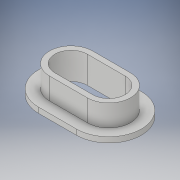
# Autodesk Inventor part: Flanec_podProvoda
Saved by Autodesk Inventor 2017 (Build 210142000, 142)
## iProperties
Part Number: Flanec_podProvoda
Material: Типовые
Document SubType Name: Modeling
Designer: Тетяна
Density: 1 g/cm^3
Appearance: По умолчанию
Author: Тетяна
Autodesk Inventor part; units mm, degrees
ref_plane "YZ Plane" through (0, 0, 0) normal (1, 0, 0) x (0, 1, 0)
ref_plane "XZ Plane" through (0, 0, 0) normal (0, 1, 0) x (-1, 0, 0)
ref_plane "XY Plane" through (0, 0, 0) normal (0, 0, 1) x (1, 0, 0)
sketch "Эскиз1" plane through (0, 0, 0) normal (0, 1, 0) x (-1, 0, 0)
  line L0 (0, 0) -> (-7, 0) construction
  line L1 (0, 4) -> (-7, 4)
  line L2 (-7, -4) -> (0, -4)
  arc A0 (0, -4) -> (0, 4) centre (0, 0) ccw
  arc A1 (-7, 4) -> (-7, -4) centre (-7, 0) ccw
  point P0 (-3.5, 0)
  dimension "d0" = 7
  dimension "d1" = 8
  constraints: 8 end point, 4 point on circle, 4 tangent, 2 centre point, 1 horizontal, 1 midpoint, 1 parallel
  measures "d0" distance of L0.start L0.end
  measures "d1" diameter of A1
extrude "Выдавливание1" add sketch "Эскиз1" along normal blind 5
sketch "Эскиз2" plane through (0, 0, 0) normal (0, -1, 0) x (1, 0, 0)
  line L0 (0, 4) -> (7, 4) projected
  arc A0 (0, 4) -> (0, -4) centre (0, 0) ccw projected
  line L1 (7, -4) -> (0, -4) projected
  arc A1 (7, -4) -> (7, 4) centre (7, 0) ccw projected
  arc A2 (0, 6) -> (0, -6) centre (0, 0) ccw
  line L2 (0, 6) -> (7, 6)
  arc A3 (7, -6) -> (7, 6) centre (7, 0) ccw
  line L3 (7, -6) -> (0, -6)
  dimension "d4" = 2
  constraints: 4 end point, 4 point on circle, 2 centre point, 3 other
  measures "d4" radial gap between concentric circles of A0 A2
extrude "Выдавливание2" add sketch "Эскиз2" against normal blind 1
sketch "Эскиз3" plane through (0, 5, 0) normal (0, 1, 0) x (1, 0, 0)
  line L0 (0, -4) -> (7, -4) projected
  arc A0 (7, -4) -> (7, 4) centre (7, 0) ccw projected
  line L1 (7, 4) -> (0, 4) projected
  arc A1 (0, 4) -> (0, -4) centre (0, 0) ccw projected
  line L2 (0, 3) -> (7, 3)
  arc A2 (7, -3) -> (7, 3) centre (7, 0) ccw
  line L3 (7, -3) -> (0, -3)
  arc A3 (0, 3) -> (0, -3) centre (0, 0) ccw
  dimension "d7" = 1
  constraints: 4 end point, 4 point on circle, 2 centre point, 3 other
  measures "d7" distance between parallel lines of L1 L2
extrude "Выдавливание3" cut sketch "Эскиз3" against normal up to surface (5 mm away) contours L2 A2 L3 A3
